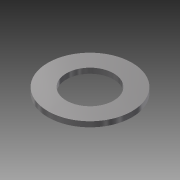
# Autodesk Inventor part: 02
Saved by Autodesk Inventor 2013 (Build 170138000, 138)
## iProperties
Created: 2014-02-07
Material: ステンレス鋼、440C
Document SubType Name: Modeling
Designer: andou
Density: 8.47 g/cm^3
Mass: 0.0665232 g
Surface Area: 0.471239 cm^2
Volume: 0.00785398 cm^3
Part Number: 02
Author: andou
Title: Bearing_Washer
Autodesk Inventor part; units mm, degrees
ref_plane "YZ Plane" through (0, 0, 0) normal (1, 0, 0) x (0, 1, 0)
ref_plane "XZ Plane" through (0, 0, 0) normal (0, 1, 0) x (-1, 0, 0)
ref_plane "XY Plane" through (0, 0, 0) normal (0, 0, 1) x (1, 0, 0)
sketch "スケッチ1" plane through (0, 0, 0) normal (0, 0, 1) x (1, 0, 0)
  circle A0 centre (0, 0) radius 4
  circle A1 centre (0, 0) radius 2.25
  dimension "d0" = 4.5
  dimension "d1" = 8
  constraints: 2 centre point, 2 coincident
  measures "d0" diameter of A1
  measures "d1" diameter of A0
extrude "押し出し1" add sketch "スケッチ1" along normal blind 0.5
